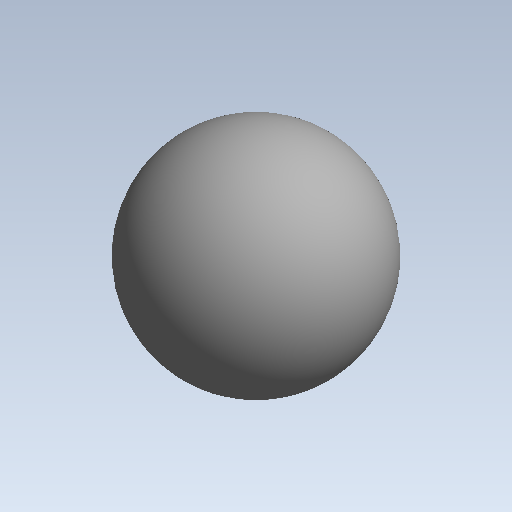
# Autodesk Inventor part: W686ZZ Ball
Saved by Autodesk Inventor 2021.3 (Build 253353010, 353A)
## iProperties
Part Number: W686ZZ Ball
Material: 一般
Catalog Web Link: www.cadenas.de
Description: Six types ball-Metric system sizes
Vendor: NTN
Document SubType Name: Modeling
Designer: partserver
Manufacturer: NTN
Mass: 0.00465766 g
Surface Area: 0.134874 cm^2
Volume: 0.00465766 cm^3
Density: 1 g/cm^3
Appearance: PSOLRGB-192-192-192
Category: PARTsolutions
Company: NTN
PSOL_IDENT_0: {$CADENAS_DATA\23d-libs\ntn\ball_roller_bearings\miniature_extra_small_bb\metric_system_sizes\mss_ba
PSOL_IDENT_1: ll.prj},173 {VTYP=3D},{NB=W686ZZ Ball},{LINA=W686ZZ Ball},{NN=Six types ball},{DATE=23.10.2020 01:13
PSOL_IDENT_2: :34},{GEOMDATE=06.03.2020 10:07:36},{VERSION=},{LINEID=12860},{WBVAR=},{WBNUMERIC=}  {NB=W686ZZ Ball
PSOL_IDENT_3: },{LINA=W686ZZ Ball},{KT=DUMMY},{IDNR=},{SD=6.0},{D=13},{B=3.5},{R=0.15},{ORDER=W686ZZ},{CR=1 080},{
PSOL_IDENT_4: COR=440},{CRF=110},{CORF=45},{LSG=39 000},{LSO=46 000},{MASS=1.90},{ORDER1=686},{D1=15.0},{D2=15.2},
PSOL_IDENT_5: {C1=1.0},{C2=1.1},{WSS=W686ZZ},{WDS=ZZ},{UTWF=FL686},{FORSS=FLW686Z},{FORDS=ZZ},{DA1=7},{DA2=7,2},{D
PSOL_IDENT_6: A=11,8},{RAS=0,15},{MASS1=2.20},{B1=5.0},{VERS=3},{X=3.5},{N=8},{O=29.83},{RB=1.036}
NB: W686ZZ Ball
NN: Six types ball
NT: Metric system sizes
NBSYN: $ORDER. Ball
LINA: W686ZZ Ball
CATALOG: NTN Corporation
SD: 6
D: 13
B: 3.5
R: 0.15
CR: 1 080
COR: 440
CRF: 110
CORF: 45
LSG: 39 000
LSO: 46 000
MASS: 1.9
ORDER1: 686
D1: 15
D2: 15.2
C1: 1
C2: 1.1
WSS: W686ZZ
WDS: ZZ
UTWF: FL686
FORSS: FLW686Z
FORDS: ZZ
DA1: 7
DA2: 7,2
DA: 11,8
RAS: 0,15
MASS1: 2.2
B1: 5
VERS: 3
SUPPLIER: NTN
ARTICLENO: W686ZZ Ball
BOMINFO: W686ZZ Ball
CREATOR: CADENAS GmbH
Title: W686ZZ Ball
Author: Cadenas PARTsolutions
Comments: Metric system sizes
Autodesk Inventor part; units mm, degrees
sketch "Sketch_1" plane through (0, 0, 0) normal (0, 0, 1) x (1, 0, 0)
  line L0 (1.036, 0) -> (-1.036, 0)
  arc A0 (1.036, 0) -> (-1.036, 0) centre (0, 0) ccw
  line L1 (1.036, 0) -> (-1.036, 0)
  constraints: 4 end point, 2 point on circle, 1 centre point
revolve "Revolution1" add sketch "Sketch_1" angle 360 about axis through (1.036, 0, 0) along (1, 0, 0)
ref_plane "mss_ball_XY" through (0, 0, 0) normal (1, 0, 0) x (0, 0, -1)
ref_plane "mss_ball_YZ" through (0, 0, 0) normal (0, 0, -1) x (0, 1, 0)
ref_plane "mss_ball_ZX" through (0, 0, 0) normal (0, 1, 0) x (1, 0, 0)
body "Solid1"
